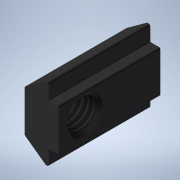
# Autodesk Inventor part: SHNTU5-5
Saved by Autodesk Inventor 2021 (Build 250183000, 183)
## iProperties
Created: 2025-07-10
Part Number: SHNTU5-5
Material: Generic
Catalog Web Link: www.cadenas.de
Description: HNTU5, HNTUV5, HNTUZ5, SHNTU5-Pre-Assembly Insertion Nuts For HFS5 Series Aluminum Extrusions 20, 25, 40 Square
Vendor: MISUMI
Document SubType Name: Modeling
Designer: psAdmin
Manufacturer: MISUMI
Mass: 0.425659 g
Surface Area: 4.84641 cm^2
Volume: 0.425659 cm^3
Density: 1 g/cm^3
Appearance: PSOLRGB-175-175-175
Category: PARTsolutions
Company: MISUMI
Title: SHNTU5-5
Author: Cadenas PARTsolutions
Comments: Pre-Assembly Insertion Nuts For HFS5 Series Aluminum Extrusions 20, 25, 40 Square
PSOL_IDENT_0: {$CADENAS_DATA/23d-libs/misumi/metric/38_al_extrusions_blackets/nuts/hntu5.prj},181 {VTYP=3D},{NB=SH
PSOL_IDENT_1: NTU5-5},{LINA=SHNTU5-5},{NN=HNTU5, HNTUV5, HNTUZ5, SHNTU5},{DATE=16.05.2023 02:30:27},{GEOMDATE=05.1
PSOL_IDENT_2: 1.2019 07:02:46},{VERSION=},{LINEID=50},{WBVAR=M},{WBNUMERIC=M}  {NB=SHNTU5-5},{LINA=SHNTU5-5},{KT=D
PSOL_IDENT_3: UMMY},{PN=SHNTU5-5},{TYPE=SHNTU5},{TS=Sintering, 304 Stainless Steel Equivalent},{M=5},{MALG=3, 4, 5
PSOL_IDENT_4: },{T=4.7},{L1=3.5},{A=5.800},{B=10},{E=3.3},{L=14},{M1=3.5},{L2=3.5}
NB: SHNTU5-5
NN: HNTU5, HNTUV5, HNTUZ5, SHNTU5
NT: Pre-Assembly Insertion Nuts For HFS5 Series Aluminum Extrusions 20, 25, 40 Square
NBSYN: $PN.
LINA: SHNTU5-5
CATALOG: Misumi
PN: SHNTU5-5
TS: Sintering, 304 Stainless Steel Equivalent
M: 5
T: 4.7
L1: 3.5
SUPPLIER: MISUMI
ARTICLENO: SHNTU5-5
BOMINFO: SHNTU5-5
CREATOR: CADENAS GmbH
Autodesk Inventor part; units mm, degrees
sketch "_____1" plane through (0, 0, 0) normal (0, 0, 1) x (1, 0, 0)
  line L0 (-4.7, 2.7981) -> (-4.7, -2.7981)
  arc A0 (-4.7, -2.7981) -> (-4.6176, -2.9599) centre (-4.5, -2.7981) ccw
  line L1 (-4.6176, -2.9599) -> (-1.8622, -4.9618)
  arc A1 (-1.8622, -4.9618) -> (-1.7446, -5) centre (-1.7446, -4.8) ccw
  line L2 (-1.7446, -5) -> (-1.6, -5)
  arc A2 (-1.6, -5) -> (-1.4, -4.8) centre (-1.6, -4.8) ccw
  line L3 (-1.4, -4.8) -> (-1.4, -3)
  arc A3 (-1.3, -2.9) -> (-1.4, -3) centre (-1.3, -3) ccw
  line L4 (-1.3, -2.9) -> (-0.2, -2.9)
  arc A4 (-0.2, -2.9) -> (0, -2.7) centre (-0.2, -2.7) ccw
  line L5 (0, -2.7) -> (0, 2.7)
  arc A5 (0, 2.7) -> (-0.2, 2.9) centre (-0.2, 2.7) ccw
  line L6 (-0.2, 2.9) -> (-1.3, 2.9)
  arc A6 (-1.4, 3) -> (-1.3, 2.9) centre (-1.3, 3) ccw
  line L7 (-1.4, 3) -> (-1.4, 4.8)
  arc A7 (-1.4, 4.8) -> (-1.6, 5) centre (-1.6, 4.8) ccw
  line L8 (-1.6, 5) -> (-1.7446, 5)
  arc A8 (-1.7446, 5) -> (-1.8622, 4.9618) centre (-1.7446, 4.8) ccw
  line L9 (-1.8622, 4.9618) -> (-4.6176, 2.9599)
  arc A9 (-4.6176, 2.9599) -> (-4.7, 2.7981) centre (-4.5, 2.7981) ccw
  constraints: 20 end point, 20 point on circle, 10 centre point
extrude "Extrusion1" add sketch "_____1" against normal blind 14
sketch "_____2" plane through (0, 0, -3.5) normal (0, 0, 1) x (1, 0, 0)
  line L0 (0, 0) -> (-4.7, 0)
  line L1 (-4.7, 0) -> (-4.7, 2.5)
  line L2 (-4.7, 2.5) -> (-4.267, 2.067)
  line L3 (-4.267, 2.067) -> (-0.433, 2.067)
  line L4 (-0.433, 2.067) -> (0, 2.5)
  line L5 (0, 2.5) -> (0, 0)
  line L6 (0, 0) -> (-4.7, 0)
  constraints: 14 end point
revolve "Revolution1" cut sketch "_____2" angle 360 about axis through (0, 0, -3.5) along (1, 0, 0)
thread "Thread1" size "M5x0.8" class "6H" standard "ISO Metric profile" full length
sketch "_____3" plane through (0, 0, -10.5) normal (0, 0, 1) x (1, 0, 0)
  line L0 (-3.65, 0) -> (-5.4, 0)
  line L1 (-5.4, 0) -> (-5.4, 1.75)
  line L2 (-5.4, 1.75) -> (-3.65, 1.75)
  line L3 (-3.65, 1.75) -> (-3.65, 0)
  line L4 (-3.65, 0) -> (-5.4, 0)
  constraints: 10 end point
revolve "Revolution2" cut sketch "_____3" angle 360 about axis through (-3.65, 0, -10.5) along (1, 0, 0)
sketch "_____4" plane through (0, 0, -10.5) normal (0, 0, 1) x (1, 0, 0)
  line L0 (-3.65, 1.75) -> (-3.65, -1.75)
  arc A0 (-3.65, 1.75) -> (-3.65, -1.75) centre (-3.65, 0) ccw
  line L1 (-3.65, 1.75) -> (-3.65, -1.75)
  constraints: 4 end point, 2 point on circle, 1 centre point
revolve "Revolution3" add sketch "_____4" angle 360 about axis through (-3.65, 1.75, -10.5) along (0, 1, 0)
ref_plane "to_blackets_XY" through (0, 0, -3.5) normal (1, 0, 0) x (0, 0, -1)
ref_plane "to_blackets_YZ" through (0, 0, -3.5) normal (0, 0, -1) x (0, 1, 0)
ref_plane "to_blackets_ZX" through (0, 0, -3.5) normal (0, 1, 0) x (1, 0, 0)
ref_plane "to_bolt_XY" through (-4.7, 0, -3.5) normal (1, 0, 0) x (0, 0, -1)
ref_plane "to_bolt_YZ" through (-4.7, 0, -3.5) normal (0, 0, -1) x (0, 1, 0)
ref_plane "to_bolt_ZX" through (-4.7, 0, -3.5) normal (0, 1, 0) x (1, 0, 0)
ref_plane "to_frames_XY" through (-1.4, 0, -3.5) normal (1, 0, 0) x (0, 0, -1)
ref_plane "to_frames_YZ" through (-1.4, 0, -3.5) normal (0, 0, -1) x (0, 1, 0)
ref_plane "to_frames_ZX" through (-1.4, 0, -3.5) normal (0, 1, 0) x (1, 0, 0)
body "Solid1"
